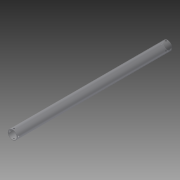
# Autodesk Inventor part: Polycarbonate Roller 1.25 OD 1.125 ID (8585K63)
Saved by Autodesk Inventor 2014 (Build 180170000, 170)
## iProperties
Created: 2014-01-12
Part Number: Polycarbonate Roller 1.25 OD 1.125 ID (8585K63)
Material: Polycarbonate, Clear
Document SubType Name: Modeling
Designer: Michael
Mass: 100.591 g
Surface Area: 1061.01 cm^2
Volume: 83.8259 cm^3
Density: 1.2 g/cm^3
Appearance: Polycarbonate - Clear
Author: Michael
Autodesk Inventor part; units mm, degrees
ref_plane "XY Plane" through (0, 0, 0) normal (0, 0, 1) x (1, 0, 0)
sketch "Sketch1" plane through (0, 0, 0) normal (0, 0, 1) x (1, 0, 0)
  circle A0 centre (0, 0) radius 15.875
  circle A1 centre (0, 0) radius 14.2875
  dimension "d0" = 31.75
  dimension "d1" = 28.575
  constraints: 2 centre point, 2 coincident
  measures "d0" diameter of A0
  measures "d1" diameter of A1
extrude "Extrusion1" add sketch "Sketch1" along normal blind 533.4
ref_plane "Work Plane1" through (0, -15.875, 0) normal (0, 1, 0) x (-1, 0, 0)
sketch "Sketch2" plane through (0, -15.875, 0) normal (0, 1, 0) x (-1, 0, 0)
  line L0 (15.875, 533.4) -> (-15.875, 533.4) projected
  line L1 (-15.875, 0) -> (15.875, 0) projected
  line L2 (18.6459, 266.7) -> (-13.1041, 266.7) construction
  line L3 (15.875, 0) -> (15.875, 533.4) construction
  line L4 (-15.875, 0) -> (-15.875, 533.4) construction
  circle A0 centre (0, 5.5563) radius 2.413
  circle A1 centre (0, 527.8438) radius 2.413
  point P0 (0, 0)
  dimension "d4" = 266.7
  dimension "d5" = 4.826
  dimension "d6" = 5.5563
  dimension "d7" = 15.875
  constraints: 2 centre point, 2 end point, 1 parallel, 1 symmetric about line, 1 other
  measures "d4" distance between parallel lines of L2 L1
  measures "d5" diameter of A0
  measures "d6" distance from line of L1 A0.centre
  measures "d7" distance from line of L3 A0.centre
extrude "Extrusion2" cut sketch "Sketch2" along normal blind 50.8
ref_plane "Work Plane2" through (15.875, 0, 0) normal (1, 0, 0) x (0, 1, 0)
sketch "Sketch3" plane through (15.875, 0, 0) normal (1, 0, 0) x (0, 1, 0)
  line L0 (-15.875, 0) -> (15.875, 0) projected
  line L1 (15.875, 0) -> (15.875, 533.4) projected
  line L2 (-15.875, 0) -> (-15.875, 533.4) projected
  line L3 (15.875, 533.4) -> (-15.875, 533.4) projected
  line L4 (15.875, 266.7) -> (-15.875, 266.7) construction
  circle A0 centre (0, 5.5563) radius 2.413
  circle A1 centre (0, 527.8438) radius 2.413
  point P0 (0, 0)
  dimension "d10" = 266.7
  dimension "d11" = 4.826
  dimension "d12" = 5.5563
  dimension "d13" = 15.875
  constraints: 2 centre point, 2 end point, 2 midpoint, 1 perpendicular, 1 symmetric about line, 1 other
  measures "d10" distance between parallel lines of L3 L4
  measures "d11" diameter of A0
  measures "d12" distance from line of L0 A0.centre
  measures "d13" distance from line of A0.centre L2
extrude "Extrusion3" cut sketch "Sketch3" against normal blind 50.8 contours A0 | A1
equation "\"d4\" = 0.5 * d2"
equation "\"d10\" = 0.5 * d2"
equation "\"d2\" = 533.4"
body "Solid1"
